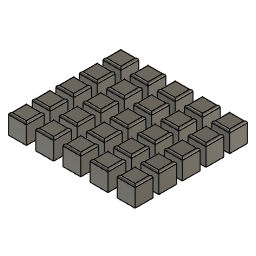
mini pad buttons (Autodesk Fusion 360 design; units mm, degrees)
Autodesk Fusion 360 part; units mm, degrees
note: some values were not read from the file. Chosen so that the rebuilt part matches the saved one: which bodies a step acts on.
sketch "Sketch1" plane through (0, 0, 0) normal (0, 0, 1) x (1, 0, 0)
  line L0 (0, 0) -> (10, 0)
  line L1 (10, 0) -> (10, 10)
  line L2 (10, 10) -> (0, 10)
  line L3 (0, 10) -> (0, 0)
  dimension "d1" = 10
  dimension "d2" = 10
  constraint horizontal L0
  constraint vertical L1
  constraint horizontal L2
  constraint vertical L3
  constraint coincident L0.start L3.end
  measures "d1" distance of L0.start L0.end
  measures "d2" distance of L0.start L2.end
extrude "Extrude1" add sketch "Sketch1" along normal blind 11 makes body 1
fillet "Fillet1" radius 1 4 edges at (10, 5, 11) (5, 0, 11) (0, 5, 11) (5, 10, 11) on bodies 1
shell "Shell1" thickness 1 removed faces 1 at (3.3333, 6.6667, 0) on bodies 1
sketch "Sketch2" plane through (0, 1, 0) normal (0, 1, 0) x (-1, 0, 0)
  line L0 (-9, 10) -> (-9, 0)
  line L1 (-9, 0) -> (-1, 0)
  line L2 (-1, 0) -> (-1, 10)
  line L3 (-1, 10) -> (-9, 10)
  line L4 (-9, 0) -> (-1, 0)
  line L5 (-1, 0) -> (-1, 2)
  line L6 (-1, 2) -> (-9, 2)
  line L7 (-9, 2) -> (-9, 0)
  dimension "d7" = 2
  constraint horizontal L4
  constraint vertical L5
  constraint horizontal L6
  constraint vertical L7
  constraint coincident L2 L5.end
  constraint coincident L0.end L1.start
  measures "d7" distance of L0.end L6.end
extrude "Extrude2" add sketch "Sketch2" along normal blind 8 contours L0 L1 L2 L4 L5 L6 L7 bodies 1
pattern_linear "R-Pattern1" count 1 spacing 0 along (0, 0, 1) count 5 spacing 13.25 along (0, 1, 0) of bodies 1 makes body 2 at (6.6667, 16.5833, 0) makes body 3 at (6.6667, 29.8333, 0) makes body 4 at (6.6667, 43.0833, 0) makes body 5 at (6.6667, 56.3333, 0)
pattern_linear "R-Pattern2" count 5 spacing 15.25 along (1, 0, 0) of bodies 3 5 2 4 1 makes body 6 at (21.9167, 3.3333, 0) makes body 7 at (30.5, 6.6667, 3.3333) makes body 8 at (52.4167, 3.3333, 0) makes body 9 at (61, 6.6667, 3.3333) makes body 10 at (21.9167, 29.8333, 0) makes body 11 at (37.1667, 29.8333, 0) makes body 12 at (52.4167, 29.8333, 0) makes body 13 at (61, 33.1667, 6.6667) makes body 14 at (21.9167, 16.5833, 0) makes body 15 at (37.1667, 16.5833, 0) makes body 16 at (52.4167, 16.5833, 0) makes body 17 at (61, 19.9167, 6.6667) makes body 18 at (21.9167, 43.0833, 0) makes body 19 at (30.5, 46.4167, 3.3333) makes body 20 at (52.4167, 43.0833, 0) makes body 21 at (61, 46.4167, 3.3333) makes body 22 at (21.9167, 56.3333, 0) makes body 23 at (30.5, 59.6667, 3.3333) makes body 24 at (52.4167, 56.3333, 0) makes body 25 at (61, 59.6667, 3.3333)
